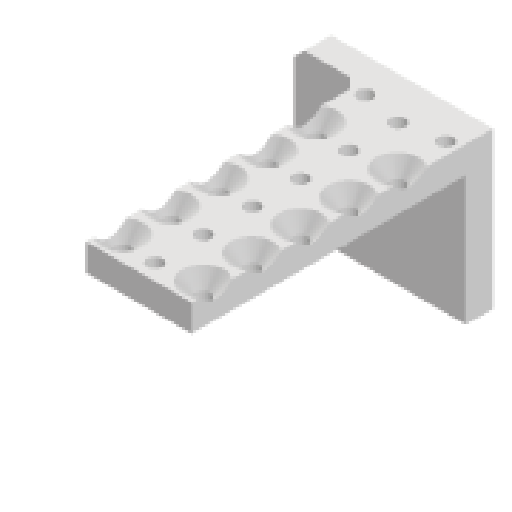
# Autodesk Inventor part: OT2-Gripper_slider
Saved by Autodesk Inventor 2024.1 (Build 281209000, 209)
## iProperties
Created: 2024-09-05
Part Number: OT2-Gripper_slider
Material: Generisch
Document SubType Name: Modeling
Designer: diederichbenedict
Density: 1 g/cm^3
Appearance: Vorgabe
Author: diederichbenedict
Autodesk Inventor part; units mm, degrees
ref_plane "YZ Plane" through (0, 0, 0) normal (1, 0, 0) x (0, 1, 0)
ref_plane "XZ Plane" through (0, 0, 0) normal (0, 1, 0) x (-1, 0, 0)
ref_plane "XY Plane" through (0, 0, 0) normal (0, 0, 1) x (1, 0, 0)
ref_plane "Arbeitsebene1" through (0, 8.4109, 0) normal (0, 0, 1) x (1, 0, 0)
sketch "Skizze1" plane through (0, 8.4109, 0) normal (0, 0, 1) x (1, 0, 0)
  line L0 (0, -27.3109) -> (0, -8.4109) projected
  line L1 (0, -27.3109) -> (4.55, -27.3109) projected
  line L2 (4.55, -27.3109) -> (4.55, -8.4109) projected
  line L3 (0, -8.4109) -> (4.55, -8.4109) projected
  circle A0 centre (2.3, -22.8609) radius 1.25 projected
  circle A1 centre (2.3, -12.8609) radius 1.25 projected
  line L4 (19.6, -27.3109) -> (19.6, -8.4109) projected
  line L5 (15.05, -8.4109) -> (19.6, -8.4109) projected
  line L6 (15.05, -27.3109) -> (15.05, -8.4109) projected
  line L7 (15.05, -27.3109) -> (19.6, -27.3109) projected
  circle A2 centre (17.3, -12.8609) radius 1.25 projected
  circle A3 centre (17.3, -22.8609) radius 1.25 projected
  line L8 (0, -8.4109) -> (19.6, -8.4109)
  line L9 (19.6, -8.4109) -> (19.6, -27.3109)
  line L10 (19.6, -27.3109) -> (0, -27.3109)
  line L11 (0, -27.3109) -> (0, -8.4109)
  line L12 (19.6, -8.4109) -> (0, -8.4109)
  line L13 (0, -8.4109) -> (0, 23.5891)
  line L14 (0, 23.5891) -> (19.6, 23.5891)
  line L15 (19.6, 23.5891) -> (19.6, -8.4109)
  line L16 (19.6, 23.5891) -> (-12.4, 23.5891)
  line L17 (-12.4, 23.5891) -> (-12.4, 28.5891)
  line L18 (-12.4, 28.5891) -> (19.6, 28.5891)
  line L19 (19.6, 28.5891) -> (19.6, 23.5891)
  point P0 (19.6, -8.4109)
  point P1 (0, 23.5891)
  point P2 (15.05, -8.4109)
  point P3 (4.55, -8.4109)
  point P4 (4.55, -27.3109)
  point P5 (0, -27.3109)
  dimension "d2" = 32
  dimension "d3" = 32
  dimension "d4" = 5
  constraints: 24 end point, 6 parallel, 3 horizontal, 3 perpendicular
  measures "d2" distance of L12.end L13.end
  measures "d3" distance of L17.end L18.end
  measures "d4" distance of L16.end L17.end
extrude "Extrusion1" add sketch "Skizze1" along normal blind 5 contours L0 L3 L2 L1 | L13 L14 L15 L5 L8 L3 | L2 L8 L6 L10 | L16 L17 L18 L19 L14 | L6 L5 L4 L7 | A1 | A2
sketch "Skizze2" plane through (-12.4, 37, 0) normal (0, 1, 0) x (1, 0, 0)
  circle A0 centre (7.1, 20.1) radius 1.4224 projected
  line L0 (32, 0) -> (0, 0) projected
  line L1 (0, 0) -> (0, -5) projected
  line L2 (32, -5) -> (0, -5) projected
  line L3 (32, 0) -> (32, -5) projected
  line L4 (0, 0) -> (32, 0)
  line L5 (32, 0) -> (32, 24)
  line L6 (32, 24) -> (0, 24)
  line L7 (0, 24) -> (0, 0)
  circle A1 centre (7.1, 20.1) radius 1.1
  point P0 (12.4, 0)
  point P1 (32, 0)
  dimension "d5" = 24
  dimension "d9" = 2.2
  constraints: 8 end point, 2 parallel, 1 centre point, 1 coincident, 1 horizontal, 1 perpendicular
  measures "d5" distance of L5.end L4.end
  measures "d9" diameter of A1
extrude "Extrusion2" add sketch "Skizze2" against normal up to surface (5 mm away) contours A0 | L0 L7 L6 L5
sketch "Skizze4" plane through (0, 8.4109, 5) normal (0, 0, 1) x (1, 0, 0)
  line L0 (9.8, -64.4629) -> (9.8, 23.7371)
  line L1 (0, -27.3109) -> (19.6, -27.3109) projected
  circle A0 centre (2.3, -22.8609) radius 1.25 projected
  circle A1 centre (17.3, -22.8609) radius 1.25 projected
  point P0 (0, -8.4109)
  point P1 (9.8, -24.3109)
  dimension "d27" = 3
  constraints: 2 end point, 1 point on line, 1 vertical, 2 other
  measures "d27" distance from line of point (9.8, -24.311) L1
hole "Bohrung1" at (9.8, -15.9, 5) at (2.3, -14.45, 5) at (17.3, -14.45, 5) direction (0, 0, -1) diameter 2.8 depth 15 tip angle 118
pattern_linear "Rechteckige Anordnung1" count 6 spacing 9 along (0, 1, 0) of "Bohrung1"
chamfer "Fasen1" distance 2 angle 45 3 edges at (0, 32, 2.5) (-12.4, 34.5, 5) (-12.4, 34.5, -24)
sketch "Skizze5" plane through (19.6, 32, -24) normal (0, -1, 0) x (1, 0, 0)
  circle A0 centre (-24.9, 3.9) radius 1.4224 projected
  circle A1 centre (-24.9, 3.9) radius 3.5
  point P0 (-19.6, 24)
  dimension "d24" = 7
  constraints: 1 centre point, 1 coincident
  measures "d24" diameter of A1
extrude "Extrusion3" cut sketch "Skizze5" against normal blind 4.3 contours A0 | A1
chamfer "Fasen3" distance 2.5 angle 45 10 edges at (17.3, -13.05, 5) (17.3, -4.05, 5) (17.3, 4.95, 5) (17.3, 13.95, 5) (17.3, 22.95, 5) (2.3, -13.05, 5) (2.3, -4.05, 5) (2.3, 4.95, 5) (2.3, 13.95, 5) (2.3, 22.95, 5)
